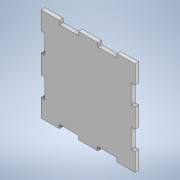
# Autodesk Inventor part: Backandfront_2
Saved by Autodesk Inventor 2020 (Build 240168000, 168)
## iProperties
Created: 2020-12-28
Part Number: Backandfront_2
Material: Generic
Document SubType Name: Modeling
Designer: solar
Density: 1 g/cm^3
Appearance: Default
Author: solar
Autodesk Inventor part; units mm, degrees
ref_plane "YZ Plane" through (0, 0, 0) normal (1, 0, 0) x (0, 1, 0)
ref_plane "XZ Plane" through (0, 0, 0) normal (0, 1, 0) x (-1, 0, 0)
ref_plane "XY Plane" through (0, 0, 0) normal (0, 0, 1) x (1, 0, 0)
sketch "Sketch1" plane through (0, 0, 0) normal (0, 0, 1) x (1, 0, 0)
  line L0 (-75, 75) -> (75, -75) construction
  line L1 (75, 75) -> (-75, -75) construction
  line L2 (0, -75) -> (15.375, -75)
  line L3 (15.375, -75) -> (15.375, -69)
  line L4 (15.375, -69) -> (46.125, -69)
  line L5 (46.125, -69) -> (46.125, -75)
  line L6 (75, -75) -> (46.125, -75)
  line L7 (75, -75) -> (75, -44.25)
  line L8 (75, 0) -> (75, -15.375)
  line L9 (75, -15.375) -> (69, -15.375)
  line L10 (69, -15.375) -> (69, -46.125)
  line L11 (69, -46.125) -> (75, -46.125)
  line L12 (75, 0) -> (75, 15.375)
  line L13 (75, 15.375) -> (69, 15.375)
  line L14 (69, 15.375) -> (69, 46.125)
  line L15 (69, 46.125) -> (75, 46.125)
  line L16 (-15.375, -75) -> (-15.375, -69)
  line L17 (-15.375, -69) -> (-46.125, -69)
  line L18 (-46.125, -69) -> (-46.125, -75)
  line L19 (-75, -75) -> (-46.125, -75)
  line L20 (-75, 15.375) -> (-69, 15.375)
  line L21 (-69, 15.375) -> (-69, 46.125)
  line L22 (-69, 46.125) -> (-75, 46.125)
  line L23 (-15.375, 75) -> (-15.375, 69)
  line L24 (-15.375, 69) -> (-46.125, 69)
  line L25 (-46.125, 69) -> (-46.125, 75)
  line L26 (15.375, 75) -> (15.375, 69)
  line L27 (15.375, 69) -> (46.125, 69)
  line L28 (46.125, 69) -> (46.125, 75)
  line L29 (-69, -46.125) -> (-75, -46.125)
  line L30 (-69, -15.375) -> (-69, -46.125)
  line L31 (-75, -15.375) -> (-69, -15.375)
  line L32 (15.375, -75) -> (-15.375, -75)
  line L33 (-46.125, -75) -> (-75, -75)
  line L34 (75, 75) -> (75, 46.125)
  line L35 (75, 15.375) -> (75, -15.375)
  line L36 (75, -46.125) -> (75, -75)
  line L37 (-75, 75) -> (-46.125, 75)
  line L38 (-75, 46.125) -> (-75, 75)
  line L39 (-75, -15.375) -> (-75, 15.375)
  line L40 (-75, -46.125) -> (-75, -75)
  line L41 (-15.375, 75) -> (15.375, 75)
  line L42 (46.125, 75) -> (75, 75)
  point P0 (0, 0)
  dimension "d0" = 150
  dimension "d1" = 150
  dimension "d2" = 15.375
  dimension "d3" = 6
  dimension "d4" = 30.75
  dimension "d8" = 15.375
  dimension "d9" = 6
  dimension "d10" = 30.75
  constraints: 86 end point, 16 perpendicular, 16 symmetric about line, 9 parallel, 4 midpoint, 2 horizontal, 1 point on line
  measures "d0" distance of L0.end L1.end
  measures "d1" distance of L1.start L0.end
  measures "d2" distance of L2.start L2.end
  measures "d3" distance of L2.end L3.end
  measures "d4" distance of L3.end L4.end
  measures "d8" distance of L8.start L8.end
  measures "d9" distance of L8.end L9.end
  measures "d10" distance of L9.end L10.end
extrude "Extrusion1" add sketch "Sketch1" along normal blind 6
body "Solid1"
